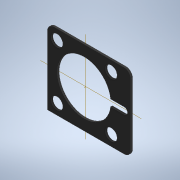
# Autodesk Inventor part: cylinder head gasket
Saved by Autodesk Inventor 2021.1 (Build 251245000, 245)
## iProperties
Created: 2020-08-30
Part Number: cylinder head gasket
Material: Rubber
Document SubType Name: Sheet Metal
Designer: Vamshi
Mass: 18.9442 g
Surface Area: 185.677 cm^2
Volume: 20.3702 cm^3
Density: 0.93 g/cm^3
Sheet Metal Rule: Default
Appearance: Rubber - Black
Author: Vamshi
Autodesk Inventor part; units mm, degrees
ref_plane "YZ Plane" through (0, 0, 0) normal (1, 0, 0) x (0, 1, 0)
ref_plane "XZ Plane" through (0, 0, 0) normal (0, 1, 0) x (-1, 0, 0)
ref_plane "XY Plane" through (0, 0, 0) normal (0, 0, 1) x (1, 0, 0)
sketch "Sketch1" plane through (0, 0, 0) normal (0, 0, 1) x (1, 0, 0)
  line L0 (-45.72, 57.15) -> (60.96, 57.15)
  line L1 (71.12, 46.99) -> (71.12, -46.99)
  line L2 (60.96, -57.15) -> (-55.88, -57.15)
  line L3 (-55.88, -57.15) -> (-55.88, 46.99)
  line L4 (-84.7488, 0) -> (99.553, 0) projected
  line L5 (0, -82.9559) -> (0, 82.9559) projected
  arc A0 (40.3212, 5.08) -> (40.3212, -5.08) centre (0, 0) ccw
  circle A1 centre (0, 0) radius 58.42 construction
  arc A2 (-45.72, 57.15) -> (-55.88, 46.99) centre (-45.72, 46.99) ccw
  arc A3 (71.12, 46.99) -> (60.96, 57.15) centre (60.96, 46.99) ccw
  arc A4 (60.96, -57.15) -> (71.12, -46.99) centre (60.96, -46.99) ccw
  line L6 (0, 0) -> (-50.4247, 50.4247) construction
  circle A5 centre (-41.3092, 41.3092) radius 8.89
  line L7 (0, 0) -> (-50.4247, -50.4247) construction
  circle A6 centre (-41.3092, -41.3092) radius 8.89
  line L8 (0, 0) -> (50.4247, -50.4247) construction
  circle A7 centre (41.3092, -41.3092) radius 8.89
  line L9 (0, 0) -> (50.4247, 50.4247) construction
  circle A8 centre (41.3092, 41.3092) radius 8.89
  arc A9 (60.96, -5.08) -> (60.96, 5.08) centre (60.96, 0) ccw
  line L10 (40.3212, 5.08) -> (60.96, 5.08)
  line L11 (40.3212, -5.08) -> (60.96, -5.08)
  point P0 (71.12, -57.15)
  point P1 (71.12, 57.15)
  point P2 (71.12, 0)
  dimension "d4" = 116.84
  dimension "d0" = 127
  dimension "d1" = 114.3
  dimension "d2" = 55.88
  dimension "d3" = 81.28
  dimension "d5" = 10.16
  dimension "d6" = 45
  dimension "d7" = 17.78
  dimension "d10" = 360
  dimension "d12" = 10.16
  dimension "d13" = 10.16
  dimension "d14" = 60.96
  constraints: 20 end point, 10 point on circle, 10 point on line, 9 centre point, 6 tangent, 3 horizontal, 2 coincident, 2 equal radius, 2 parallel, 1 horizontal alignment, 1 midpoint, 1 perpendicular, 25 other
  measures "d0" distance of point (71.12, -57.15) L2.end
  measures "d1" distance of point (71.12, 57.15) point (71.12, -57.15)
  measures "d2" distance between parallel lines of L5 L3
  measures "d3" diameter of A0
  measures "d5" radius of A2
  measures "d6" angle of L4 L6
  measures "d7" diameter of A5
  measures "d12" diameter of A9
  measures "d13" distance between parallel lines of L11 L10
  measures "d14" distance of A9.centre point (0, 0)
extrude "Extrusion1" add sketch "Sketch1" along normal blind 2.54 contours L0 L5 A0 L4 L3 A2 | L0 A3 L1 L4 A9 L10 A0 L5 | L4 A0 L5 L2 L3 | L1 A4 L2 L5 A0 L11 A9 L4
equation "\"BendRadius\" = Thickness"
equation "\"BendReliefWidth\" = Thickness"
equation "\"BendReliefDepth\" = 0.5 * Thickness"
equation "\"CornerReliefSize\" = 4 * Thickness"
equation "\"MinimumRemnant\" = 2 * Thickness"
equation "\"TransitionRadius\" = BendRadius"
equation "\"JacobiRadiusSize\" = BendRadius"
equation "\"GapSize\" = Thickness"
equation "\"Thickness\" = 3.048"
body "Solid1"
